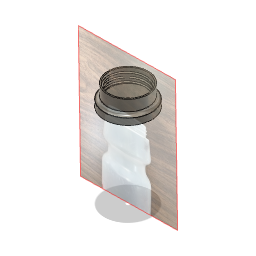
WaterBottleCap_09162021_1417 (Autodesk Fusion 360 design; units mm, degrees)
Autodesk Fusion 360 part; units mm, degrees
note: some values were not read from the file. Set by a fixed rule: which face or edge a step refers to.
sketch "Sketch1" plane through (0, 0, 0) normal (0, 1, 0) x (1, 0, 0)
  circle A0 centre (0, 0) radius 35
  dimension "d1" = 70
  constraint coincident A0.centre origin
  measures "d1" diameter of A0
sketch "Sketch2" plane through (0, 0, 0) normal (0, 0, 1) x (1, 0, 0)
sketch "Sketch3" plane through (0, 0, 0) normal (0, 0, 1) x (1, 0, 0)
sketch "Sketch4" plane through (0, 0, 0) normal (0, 0, 1) x (1, 0, 0)
sketch "Sketch5" plane through (0, 0, 0) normal (0, 0, 1) x (1, 0, 0)
sketch "Sketch6" plane through (0, 0, 0) normal (0, 0, 1) x (1, 0, 0)
sketch "Sketch7" plane through (0, 0, 0) normal (0, 1, 0) x (1, 0, 0)
sketch "Sketch8" plane through (0, 0, 0) normal (0, 1, 0) x (1, 0, 0)
  circle A0 centre (0, 0) radius 35
  dimension "d5" = 70
  constraint coincident A0.centre origin
  measures "d5" diameter of A0
surface "Extrude2" add extruded along (0, 1, 0) between 0 and 15 profiles "Sketch8" section 1 makes body 1
sketch "Sketch9" plane through (0, 0, 0) normal (0, 1, 0) x (1, 0, 0)
  circle A0 centre (0, 0) radius 30
  dimension "d8" = 60
  constraint coincident A0.centre origin
  measures "d8" diameter of A0
extrude "Extrude3" add sketch "Sketch9" along normal blind 15 separate body makes body 2
delete_face "SurfaceDeleteFace1" leaving the opening 1 faces at (-34.8261, 5, -3.4849) on bodies 1
shell "Shell2" thickness 2 outward yes removed faces 1 at (7.6631, 15, -11.2397) on bodies 2
extrude "Extrude4" cut 1 faces at (7.6631, 0, -11.2397) along direction (0, -1, 0) blind 30 on bodies 2 bodies 2
sketch "Sketch10" plane through (0, -2, 0) normal (0, -1, 0) x (1, 0, 0)
  circle A0 centre (0, 0) radius 30
  circle A1 centre (0, 0) radius 32
  dimension "d14" = 60
  dimension "d15" = 2
  dimension "d16" = 64
  measures "d14" diameter of A0
  measures "d15" distance of A0 A1
  measures "d16" diameter of A1
sketch "Sketch11" plane through (0, -2, 0) normal (0, -1, 0) x (1, 0, 0)
coil "CoilPrimitive1" add diameter 60 section triangle in size 4 on centre turns 3 pitch 6.5 right hand placed x (1, 0, 0) y (0, 0, -1) z (0, 1, 0) at (0, 0, 0) separate body makes body 3
extrude "Extrude5" add 1 faces at (31.1025, 15, -3.0802) along direction (0, 1, 0) blind 7 on bodies 2 bodies 2 3
sketch "Sketch13" plane through (0, 0, 0) normal (0, 1, 0) x (1, 0, 0)
  circle A0 centre (0, 0) radius 37.5
  dimension "d24" = 75
  constraint coincident A0.centre origin
  measures "d24" diameter of A0
extrude "Extrude6" add sketch "Sketch13" against normal blind 10 bodies 2
fillet "Fillet1" radius 5 1 edges at (-29.8345, 0, 11.5717) on bodies 2
sketch "Sketch14" plane through (0, 0, 0) normal (0, 1, 0) x (-1, 0, 0)
  spline S0 degree 3 poles (-13.1734, -26.9529) (-16.3248, -25.1725) (-19.127, -22.8356) (-23.6893, -17.3194) (-25.4322, -14.2051) (-27.742, -7.3607) (-28.2352, -3.6753) (-28, 0) knots -3.250332 -3.250332 -3.250332 -3.250332 -2.165933 -2.165933 -1.104846 -1.104846 0 0 0 0
  arc A0 (-13.1734, -26.9529) -> (-30, 0) centre (0, 0) ccw
  line L0 (-30, 0) -> (-28, 0)
  circle A1 centre (0, 0) radius 2.5
  dimension "d29" = 5
  constraint coincident A0.centre A1.centre
  measures "d29" diameter of A1
extrude "Extrude7" cut sketch "Sketch14" against normal blind 38 contours A1 bodies 2
